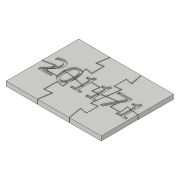
# Autodesk Inventor part: JigsawRainer
Saved by Autodesk Inventor 2019.4 (Build 234330000, 330)
## iProperties
Created: 2020-11-12
Part Number: JigsawRainer
Material: Generic
Document SubType Name: Modeling
Designer: diederichbenedict
Density: 1 g/cm^3
Appearance: Default
Author: diederichbenedict
Autodesk Inventor part; units mm, degrees
ref_plane "YZ Plane" through (0, 0, 0) normal (1, 0, 0) x (0, 1, 0)
ref_plane "XZ Plane" through (0, 0, 0) normal (0, 1, 0) x (-1, 0, 0)
ref_plane "XY Plane" through (0, 0, 0) normal (0, 0, 1) x (1, 0, 0)
sketch "Sketch1" plane through (0, 0, 0) normal (0, 1, 0) x (-1, 0, 0)
  line L0 (0, 0) -> (93.1343, 0) construction
  line L1 (93.1343, 0) -> (93.1343, -69.0996) construction
  line L2 (93.1343, -69.0996) -> (0, -69.0996) construction
  line L3 (0, -69.0996) -> (0, 0) construction
  line L4 (89.2897, -1.1317) -> (89.2897, -33.2216)
  line L5 (89.2897, -33.2216) -> (79.3554, -35.2084)
  line L6 (79.3554, -35.2084) -> (80.0913, -27.9233)
  line L7 (80.0913, -27.9233) -> (70.0834, -27.9233)
  line L8 (70.0834, -27.9233) -> (71.1872, -35.7971)
  line L9 (71.1872, -35.7971) -> (61.1602, -34.341)
  line L10 (61.1602, -34.341) -> (59.9154, -23.1337)
  line L11 (59.9154, -23.1337) -> (66.0348, -24.0224)
  line L12 (66.0348, -24.0224) -> (66.0348, -11.6508)
  line L13 (66.0348, -11.6508) -> (59.4499, -12.5739)
  line L14 (59.4499, -12.5739) -> (61.0309, -1.6875)
  line L15 (89.2897, -1.1317) -> (61.0309, -1.1317)
  line L16 (61.0309, -1.1317) -> (61.0309, -1.6875)
  line L17 (89.4151, -33.8484) -> (89.4151, -66.9252)
  line L18 (89.4151, -66.9252) -> (61.0309, -66.6319)
  line L19 (61.0309, -66.6319) -> (62.7424, -55.5046)
  line L20 (62.7424, -55.5046) -> (56.8144, -56.6902)
  line L21 (56.8144, -56.6902) -> (56.8144, -46.1474)
  line L22 (56.8144, -46.1474) -> (62.7424, -47.0592)
  line L23 (62.7424, -47.0592) -> (61.3608, -34.6937)
  line L24 (61.3608, -34.6937) -> (71.7003, -36.284)
  line L25 (71.7003, -36.284) -> (70.6353, -28.2553)
  line L26 (70.6353, -28.2553) -> (79.7233, -28.2553)
  line L27 (79.7233, -28.2553) -> (78.9055, -36.284)
  line L28 (78.9055, -36.284) -> (89.4151, -33.8484)
  line L29 (60.5378, -1.1317) -> (58.7825, -12.9338)
  line L30 (58.7825, -12.9338) -> (65.5845, -11.9802)
  line L31 (65.5845, -11.9802) -> (65.5845, -23.578)
  line L32 (65.5845, -23.578) -> (59.2997, -22.5908)
  line L33 (59.2997, -22.5908) -> (60.7075, -34.0174)
  line L34 (60.7075, -34.0174) -> (49.7501, -31.7837)
  line L35 (49.7501, -31.7837) -> (50.4751, -38.3109)
  line L36 (50.4751, -38.3109) -> (42.307, -38.3109)
  line L37 (42.307, -38.3109) -> (42.7923, -31.8702)
  line L38 (42.7923, -31.8702) -> (32.4642, -33.7719)
  line L39 (32.4642, -33.7719) -> (34.0347, -21.9149)
  line L40 (34.0347, -21.9149) -> (28.0705, -22.751)
  line L41 (28.0705, -22.751) -> (28.0705, -12.544)
  line L42 (28.0705, -12.544) -> (34.5683, -13.5648)
  line L43 (34.5683, -13.5648) -> (32.2791, -1.1317)
  line L44 (32.2791, -1.1317) -> (60.5378, -1.1317)
  line L45 (31.7936, -1.1317) -> (34.0041, -13.1375)
  line L46 (34.0041, -13.1375) -> (27.8516, -12.2224)
  line L47 (27.8516, -12.2224) -> (27.8516, -23.2571)
  line L48 (27.8516, -23.2571) -> (33.758, -22.3058)
  line L49 (33.758, -22.3058) -> (32.2292, -33.8484)
  line L50 (32.2292, -33.8484) -> (21.4646, -35.7971)
  line L51 (21.4646, -35.7971) -> (22.2468, -28.0771)
  line L52 (22.2468, -28.0771) -> (13.1675, -28.0771)
  line L53 (13.1675, -28.0771) -> (14.025, -35.7971)
  line L54 (14.025, -35.7971) -> (3.5413, -33.9813)
  line L55 (3.5413, -33.9813) -> (3.3479, -1.1317)
  line L56 (3.3479, -1.1317) -> (31.7936, -1.1317)
  line L57 (60.5332, -66.5561) -> (62.3448, -56.0974)
  line L58 (62.3448, -56.0974) -> (56.4286, -57.1685)
  line L59 (56.4286, -57.1685) -> (56.1989, -45.1765)
  line L60 (56.1989, -45.1765) -> (62.234, -46.4067)
  line L61 (62.234, -46.4067) -> (60.7871, -34.663)
  line L62 (60.7871, -34.663) -> (50.2374, -32.2665)
  line L63 (50.2374, -32.2665) -> (51.0416, -38.7929)
  line L64 (51.0416, -38.7929) -> (41.689, -38.7929)
  line L65 (41.689, -38.7929) -> (42.3502, -32.2665)
  line L66 (42.3502, -32.2665) -> (32.361, -34.5512)
  line L67 (32.361, -34.5512) -> (30.5659, -46.4067)
  line L68 (30.5659, -46.4067) -> (36.5273, -45.6723)
  line L69 (36.5273, -45.6723) -> (36.5273, -57.1685)
  line L70 (36.5273, -57.1685) -> (30.9276, -55.8964)
  line L71 (30.9276, -55.8964) -> (32.8573, -66.5561)
  line L72 (32.8573, -66.5561) -> (60.5332, -66.5561)
  line L73 (32.361, -66.5561) -> (3.3479, -66.5561)
  line L74 (3.3479, -66.5561) -> (3.3479, -34.4027)
  line L75 (3.3479, -34.4027) -> (14.4258, -36.0308)
  line L76 (14.4258, -36.0308) -> (13.3796, -28.5442)
  line L77 (13.3796, -28.5442) -> (21.8557, -28.5442)
  line L78 (21.8557, -28.5442) -> (21.0654, -36.284)
  line L79 (21.0654, -36.284) -> (31.8925, -34.4027)
  line L80 (31.8925, -34.4027) -> (30.054, -46.912)
  line L81 (30.054, -46.912) -> (36.2972, -46.0395)
  line L82 (36.2972, -46.0395) -> (36.2972, -56.5324)
  line L83 (36.2972, -56.5324) -> (30.054, -55.6149)
  line L84 (30.054, -55.6149) -> (32.361, -66.5561)
  constraints: 162 end point, 22 perpendicular, 17 parallel, 7 point on line, 3 vertical, 2 horizontal, 2 other
extrude "Extrusion1" add sketch "Sketch1" along normal blind 4
sketch "Sketch2" plane through (0, 4, 0) normal (0, 1, 0) x (1, 0, 0)
  line L0 (-85.9248, 43.9999) -> (-3.2001, 43.9999) construction
  line L1 (-3.2001, 43.9999) -> (-3.2001, 21.6179) construction
  line L2 (-3.2001, 21.6179) -> (-85.9248, 21.6179) construction
  line L3 (-85.9248, 21.6179) -> (-85.9248, 43.9999) construction
  line L4 (-73.2541, 25.2394) -> (-84.5848, 25.2394)
  line L5 (-84.5848, 25.2394) -> (-84.5848, 27.845)
  spline S0 degree 2 poles (-84.5848, 27.845) (-83.3639, 28.9915) (-81.19, 31.1206) (-80.1478, 32.2671) knots 0 0 0 1 2 2 2
  spline S1 degree 2 poles (-80.1478, 32.2671) (-78.0484, 34.575) (-76.5148, 37.3444) (-76.5148, 38.8184) knots 0 0 0 1 2 2 2
  spline S2 degree 2 poles (-76.5148, 38.8184) (-76.5148, 39.5926) (-76.9913, 40.754) (-77.4231, 41.1262) knots 0 0 0 1 2 2 2
  spline S3 degree 2 poles (-77.4231, 41.1262) (-77.8548, 41.4985) (-78.9864, 41.8707) (-79.6713, 41.8707) knots 0 0 0 1 2 2 2
  spline S4 degree 2 poles (-79.6713, 41.8707) (-80.3265, 41.8707) (-81.6665, 41.5431) (-82.277, 41.29) knots 0 0 0 1 2 2 2
  spline S5 degree 2 poles (-82.277, 41.29) (-82.7981, 41.0816) (-83.7659, 40.486) (-84.0637, 40.2775) knots 0 0 0 1 2 2 2
  line L6 (-84.0637, 40.2775) -> (-84.1977, 40.2775)
  line L7 (-84.1977, 40.2775) -> (-84.1977, 42.8981)
  spline S6 degree 2 poles (-84.1977, 42.8981) (-83.4383, 43.2703) (-80.7136, 43.9999) (-79.4927, 43.9999) knots 0 0 0 1 2 2 2
  spline S7 degree 2 poles (-79.4927, 43.9999) (-76.9168, 43.9999) (-74.0134, 41.2751) (-74.0134, 38.9524) knots 0 0 0 1 2 2 2
  spline S8 degree 2 poles (-74.0134, 38.9524) (-74.0134, 37.8655) (-74.5196, 36.049) (-74.9663, 35.2748) knots 0 0 0 1 2 2 2
  spline S9 degree 2 poles (-74.9663, 35.2748) (-75.413, 34.4707) (-76.7084, 32.8925) (-77.4231, 32.1331) knots 0 0 0 1 2 2 2
  spline S10 degree 2 poles (-77.4231, 32.1331) (-78.5844, 30.8675) (-81.4283, 28.1577) (-82.277, 27.3686) knots 0 0 0 1 2 2 2
  line L8 (-82.277, 27.3686) -> (-73.2541, 27.3686)
  line L9 (-73.2541, 27.3686) -> (-73.2541, 25.2394)
  spline S11 degree 2 poles (-59.3624, 34.4261) (-59.3624, 29.4828) (-62.236, 24.8523) (-65.2288, 24.8523) knots 0 0 0 1 2 2 2
  spline S12 degree 2 poles (-65.2288, 24.8523) (-68.2662, 24.8523) (-71.11, 29.5722) (-71.11, 34.4112) knots 0 0 0 1 2 2 2
  spline S13 degree 2 poles (-71.11, 34.4112) (-71.11, 39.3842) (-68.2364, 43.985) (-65.2288, 43.985) knots 0 0 0 1 2 2 2
  spline S14 degree 2 poles (-65.2288, 43.985) (-62.2062, 43.985) (-59.3624, 39.2204) (-59.3624, 34.4261) knots 0 0 0 1 2 2 2
  spline S15 degree 2 poles (-62.5189, 28.8277) (-62.1616, 29.7359) (-61.8638, 32.5351) (-61.8638, 34.4261) knots 0 0 0 1 2 2 2
  spline S16 degree 2 poles (-61.8638, 34.4261) (-61.8638, 36.317) (-62.1616, 39.1013) (-62.5338, 40.0393) knots 0 0 0 1 2 2 2
  spline S17 degree 2 poles (-62.5338, 40.0393) (-62.906, 40.9773) (-64.2014, 41.9451) (-65.2288, 41.9451) knots 0 0 0 1 2 2 2
  spline S18 degree 2 poles (-65.2288, 41.9451) (-66.2561, 41.9451) (-67.5813, 40.9773) (-67.9684, 40.0095) knots 0 0 0 1 2 2 2
  spline S19 degree 2 poles (-67.9684, 40.0095) (-68.3406, 39.0715) (-68.6086, 36.2128) (-68.6086, 34.4112) knots 0 0 0 1 2 2 2
  spline S20 degree 2 poles (-68.6086, 34.4112) (-68.6086, 32.4756) (-68.3704, 29.8848) (-67.9833, 28.8724) knots 0 0 0 1 2 2 2
  spline S21 degree 2 poles (-67.9833, 28.8724) (-67.6259, 27.9195) (-66.3008, 26.8921) (-65.2288, 26.8921) knots 0 0 0 1 2 2 2
  spline S22 degree 2 poles (-65.2288, 26.8921) (-64.2163, 26.8921) (-62.8911, 27.8599) (-62.5189, 28.8277) knots 0 0 0 1 2 2 2
  line L10 (-46.6023, 25.2394) -> (-55.5656, 25.2394)
  line L11 (-55.5656, 25.2394) -> (-55.5656, 27.1154)
  line L12 (-55.5656, 27.1154) -> (-52.2304, 27.1154)
  line L13 (-52.2304, 27.1154) -> (-52.2304, 39.4289)
  line L14 (-52.2304, 39.4289) -> (-55.5656, 39.4289)
  line L15 (-55.5656, 39.4289) -> (-55.5656, 41.1113)
  spline S23 degree 2 poles (-55.5656, 41.1113) (-53.6747, 41.1113) (-51.888, 42.1834) (-51.7689, 43.6723) knots 0 0 0 1 2 2 2
  line L16 (-51.7689, 43.6723) -> (-49.863, 43.6723)
  line L17 (-49.863, 43.6723) -> (-49.863, 27.1154)
  line L18 (-49.863, 27.1154) -> (-46.6023, 27.1154)
  line L19 (-46.6023, 27.1154) -> (-46.6023, 25.2394)
  line L20 (-32.8148, 25.2394) -> (-41.7782, 25.2394)
  line L21 (-41.7782, 25.2394) -> (-41.7782, 27.1154)
  line L22 (-41.7782, 27.1154) -> (-38.443, 27.1154)
  line L23 (-38.443, 27.1154) -> (-38.443, 39.4289)
  line L24 (-38.443, 39.4289) -> (-41.7782, 39.4289)
  line L25 (-41.7782, 39.4289) -> (-41.7782, 41.1113)
  spline S24 degree 2 poles (-41.7782, 41.1113) (-39.8872, 41.1113) (-38.1005, 42.1834) (-37.9814, 43.6723) knots 0 0 0 1 2 2 2
  line L26 (-37.9814, 43.6723) -> (-36.0756, 43.6723)
  line L27 (-36.0756, 43.6723) -> (-36.0756, 27.1154)
  line L28 (-36.0756, 27.1154) -> (-32.8148, 27.1154)
  line L29 (-32.8148, 27.1154) -> (-32.8148, 25.2394)
  line L30 (-17.8958, 40.8582) -> (-25.8467, 25.2394)
  line L31 (-25.8467, 25.2394) -> (-28.4672, 25.2394)
  line L32 (-28.4672, 25.2394) -> (-20.0696, 41.4538)
  line L33 (-20.0696, 41.4538) -> (-29.5541, 41.4538)
  line L34 (-29.5541, 41.4538) -> (-29.5541, 43.6127)
  line L35 (-29.5541, 43.6127) -> (-17.8958, 43.6127)
  line L36 (-17.8958, 43.6127) -> (-17.8958, 40.8582)
  line L37 (-5.2399, 25.2394) -> (-14.2033, 25.2394)
  line L38 (-14.2033, 25.2394) -> (-14.2033, 27.1154)
  line L39 (-14.2033, 27.1154) -> (-10.8681, 27.1154)
  line L40 (-10.8681, 27.1154) -> (-10.8681, 39.4289)
  line L41 (-10.8681, 39.4289) -> (-14.2033, 39.4289)
  line L42 (-14.2033, 39.4289) -> (-14.2033, 41.1113)
  spline S25 degree 2 poles (-14.2033, 41.1113) (-12.3123, 41.1113) (-10.5256, 42.1834) (-10.4065, 43.6723) knots 0 0 0 1 2 2 2
  line L43 (-10.4065, 43.6723) -> (-8.5007, 43.6723)
  line L44 (-8.5007, 43.6723) -> (-8.5007, 27.1154)
  line L45 (-8.5007, 27.1154) -> (-5.2399, 27.1154)
  line L46 (-5.2399, 27.1154) -> (-5.2399, 25.2394)
  point P0 (0, 0)
  constraints: 2 other
extrude "Extrusion2" cut sketch "Sketch2" against normal blind 1
body "Solid1"
